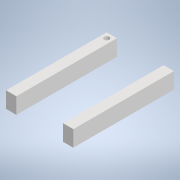
# Autodesk Inventor part: motor mount layer
Saved by Autodesk Inventor 2022 (Build 260153000, 153)
## iProperties
Created: 2021-11-30
Part Number: motor mount layer
Material: Generic
Document SubType Name: Modeling
Designer: a-dubs
Density: 1 g/cm^3
Appearance: Default
Author: a-dubs
Autodesk Inventor part; units mm, degrees
ref_plane "YZ Plane" through (0, 0, 0) normal (1, 0, 0) x (0, 1, 0)
ref_plane "XZ Plane" through (0, 0, 0) normal (0, 1, 0) x (-1, 0, 0)
ref_plane "XY Plane" through (0, 0, 0) normal (0, 0, 1) x (1, 0, 0)
sketch "Sketch1" plane through (0, 0, 0) normal (0, 1, 0) x (-1, 0, 0)
  line L0 (0, 0) -> (61, 0)
  circle A0 centre (0, 0) radius 33.6
  line L1 (61, 8.05) -> (61, 13.05)
  line L2 (72.05, 0) -> (77.05, 0)
  line L3 (61, 0) -> (61, 60)
  line L4 (0, 0) -> (-42.65, 0)
  line L5 (-42.65, 0) -> (-47.65, 0)
  line L6 (-47.65, 0) -> (-53.85, 0)
  line L7 (0, 0) -> (0, -33.6)
  line L8 (0, 0) -> (42.65, 0)
  line L9 (35.9999, 0) -> (29.9999, 0)
  line L10 (29.9999, 0) -> (29.9999, -31.3)
  line L11 (29.9999, -31.3) -> (29.9999, -37.5)
  line L12 (29.9999, -37.5) -> (78.3499, -37.5)
  line L13 (78.3499, 37.4) -> (29.9999, 37.4)
  line L14 (29.9999, 37.4) -> (29.9999, 0)
  line L15 (42.65, 31.2) -> (45.65, 31.2)
  line L16 (78.3499, 37.4) -> (82.5499, 37.4)
  line L17 (82.5499, 37.4) -> (82.5499, -37.5)
  line L18 (82.5499, -37.5) -> (78.3499, -37.5)
  line L19 (29.9999, 37.4) -> (36.3999, 37.4)
  line L20 (61, 0) -> (40, 0)
  line L21 (40, 0) -> (40, 37.4)
  line L22 (40, 0) -> (40, -37.5)
  line L23 (36.8, -37.4) -> (43.2, -37.4)
  line L24 (43.2, -37.4) -> (43.2, 37.4)
  line L25 (43.2, 37.4) -> (36.8, 37.4)
  line L26 (36.8, 37.4) -> (36.8, -37.4)
  line L27 (36.8, -37.4) -> (43.2, 37.4) construction
  line L28 (43.2, -37.4) -> (36.8, 37.4) construction
  line L29 (61, 0) -> (75.45, 0)
  line L30 (61, 0) -> (61, -18.5)
  line L31 (75.45, 18.5) -> (75.45, -18.5)
  line L32 (75.45, -18.5) -> (46.55, -18.5)
  line L33 (46.55, -18.5) -> (46.55, 18.5)
  line L34 (46.55, 18.5) -> (75.45, -18.5) construction
  line L35 (75.45, 18.5) -> (46.55, -18.5) construction
  line L36 (46.55, 18.5) -> (46.55, 37.4)
  line L37 (75.45, 18.5) -> (75.45, 37.4)
  line L38 (75.45, -18.5) -> (75.45, -37.5)
  line L39 (46.55, -18.5) -> (46.55, -37.5)
  line L40 (75.45, 18.5) -> (75.45, 28.1)
  circle A1 centre (75.45, 28.1) radius 1.6
  circle A2 centre (46.55, 28.1) radius 1.6
  line L41 (75.45, -18.5) -> (75.45, -28.1)
  circle A3 centre (75.45, -28.1) radius 1.6
  circle A4 centre (46.55, -28.1) radius 1.6
  line L42 (75.45, 28.1) -> (75.45, 31.3)
  line L43 (75.45, 31.3) -> (29.9999, 31.3)
  line L44 (75.45, -28.1) -> (75.45, -31.3)
  line L45 (75.45, -31.3) -> (29.9999, -31.3)
  line L46 (75.45, -28.1) -> (75.45, -24.9)
  line L47 (75.45, -24.9) -> (29.9999, -24.9)
  line L48 (46.55, 28.1) -> (40, 28.1)
  circle A5 centre (40, 28.1) radius 1.6
  line L49 (46.55, -28.1) -> (40, -28.1)
  circle A6 centre (40, -28.1) radius 1.6
  line L50 (75.45, 28.1) -> (75.45, 24.9)
  line L51 (75.45, 24.9) -> (29.9999, 24.9)
  line L52 (75.45, 31.3) -> (78.65, 31.3)
  line L53 (78.65, 31.3) -> (78.65, -31.3)
  line L54 (78.65, -31.3) -> (75.45, -31.3)
  line L55 (75.45, -31.3) -> (72.25, -31.3)
  line L56 (72.25, -31.3) -> (72.25, 31.3)
  line L57 (46.55, 28.1) -> (49.75, 28.1)
  line L58 (49.75, 31.3) -> (49.75, -37.5)
  circle A7 centre (75.45, -18.5) radius 1.6
  circle A8 centre (46.55, -18.5) radius 1.6
  line L59 (46.55, 18.5) -> (46.55, 21.7)
  line L60 (75.45, 18.5) -> (75.45, 13.7)
  line L61 (75.45, 13.7) -> (78.65, 13.7)
  line L62 (78.65, 13.7) -> (36.8, 13.7)
  line L63 (75.45, -18.5) -> (75.45, -21.7)
  line L64 (75.45, -21.7) -> (36.8, -21.7)
  line L65 (75.45, -21.7) -> (78.65, -21.7)
  line L66 (75.45, -18.5) -> (75.45, -13.7)
  line L67 (75.45, -13.7) -> (78.65, -13.7)
  line L68 (75.45, -13.7) -> (36.8, -13.7)
  line L69 (57.8, -13.7) -> (64.2, -13.7)
  line L70 (64.2, -13.7) -> (64.2, 13.7)
  line L71 (64.2, 13.7) -> (57.8, 13.7)
  line L72 (57.8, 13.7) -> (57.8, -13.7)
  line L73 (57.8, -13.7) -> (64.2, 13.7) construction
  line L74 (64.2, -13.7) -> (57.8, 13.7) construction
  line L75 (49.75, -3.2) -> (72.25, -3.2)
  line L76 (72.25, -3.2) -> (72.25, 3.2)
  line L77 (72.25, 3.2) -> (49.75, 3.2)
  line L78 (49.75, 3.2) -> (49.75, -3.2)
  line L79 (49.75, -3.2) -> (72.25, 3.2) construction
  line L80 (72.25, -3.2) -> (49.75, 3.2) construction
  line L81 (49.75, 3.2) -> (43.2, 3.2)
  line L82 (49.75, -3.2) -> (43.2, -3.2)
  line L83 (52.2, -8.45) -> (69.8, -8.45)
  line L84 (69.8, -8.45) -> (69.8, 8.45)
  line L85 (69.8, 8.45) -> (52.2, 8.45)
  line L86 (52.2, 8.45) -> (52.2, -8.45)
  line L87 (52.2, -8.45) -> (69.8, 8.45) construction
  line L88 (69.8, -8.45) -> (52.2, 8.45) construction
  line L89 (61, 0) -> (61, 22.2)
  line L90 (61, 22.2) -> (46.55, 22.2)
  line L91 (61, 22.2) -> (61, 17.4)
  line L92 (61, 17.4) -> (36.8, 17.4)
  line L93 (61, 22.2) -> (61, 25.4)
  line L94 (61, 25.4) -> (36.8, 25.4)
  line L95 (61, 25.4) -> (78.65, 25.4)
  line L96 (61, 17.4) -> (78.65, 17.4)
  line L97 (61, 22.2) -> (82.5499, 22.2)
  line L98 (46.55, 22.2) -> (36.8, 22.2)
  line L99 (61, 0) -> (61, -14.8)
  line L100 (61, -14.8) -> (61, -18)
  line L101 (61, -14.8) -> (61, -10)
  line L102 (61, -10) -> (36.8, -10)
  line L103 (61, -18) -> (36.8, -18)
  line L104 (61, -18) -> (82.5499, -18)
  line L105 (61, -10) -> (82.5499, -10)
  line L106 (64.2, 13.7) -> (64.2, 17.4)
  line L107 (57.8, 17.4) -> (57.8, 13.7)
  point P0 (36.8, 31.3)
  point P1 (36.8, -31.3)
  point P2 (43.2, -31.3)
  point P3 (43.2, 31.3)
  point P4 (43.2, -21.7)
  point P5 (72.25, -21.7)
  point P6 (43.2, 13.7)
  point P7 (72.25, 13.7)
  point P8 (72.25, -13.7)
  point P9 (43.2, -13.7)
  point P10 (57.8, -3.2)
  point P11 (64.2, -3.2)
  point P12 (64.2, 3.2)
  point P13 (57.8, 3.2)
  point P14 (57.8, 8.45)
  point P15 (64.2, 8.45)
  point P16 (52.2, -3.2)
  point P17 (52.2, 3.2)
  point P18 (61, 18.5)
  point P19 (72.25, 22.2)
  point P20 (46.55, 24.9)
  point P21 (43.2, 24.9)
  point P22 (43.2, 22.2)
  point P23 (72.25, -18)
  point P24 (72.25, -10)
  point P25 (64.2, -10)
  point P26 (64.2, -8.45)
  point P27 (57.8, -8.45)
  point P28 (57.8, -10)
  point P29 (43.2, -10)
  point P30 (43.2, -18)
  point P31 (72.25, 17.4)
  point P32 (72.25, 24.9)
  point P33 (43.2, 17.4)
  dimension "d1" = 67.2
  dimension "d0" = 61
  dimension "d7" = 5
  dimension "d8" = 5
  dimension "d11" = 60
  dimension "d13" = 42.65
  dimension "d14" = 5
  dimension "d15" = 6.2
  dimension "d26" = 6
  dimension "d27" = 6.2
  dimension "d42" = 3
  dimension "d46" = 4.2
  dimension "d53" = 6.4
  dimension "d54" = 21
  dimension "d55" = 6.4
  dimension "d56" = 14.45
  dimension "d57" = 18.5
  dimension "d58" = 9.6
  dimension "d60" = 3.2
  dimension "d61" = 3.2
  dimension "d62" = 3.2
  dimension "d63" = 3.2
  dimension "d64" = 3.2
  dimension "d66" = 3.2
  dimension "d67" = 3.2
  dimension "d68" = 3.2
  dimension "d69" = 3.2
  dimension "d70" = 3.2
  dimension "d71" = 3.2
  dimension "d74" = 3.2
  dimension "d75" = 3.2
  dimension "d78" = 3.2
  dimension "d79" = 4.8
  dimension "d80" = 3.2
  dimension "d81" = 4.8
  dimension "d85" = 6.4
  dimension "d86" = 6.4
  dimension "d87" = 17.6
  dimension "d88" = 16.9
  dimension "d89" = 22.2
  dimension "d90" = 4.8
  dimension "d91" = 3.2
  dimension "d92" = 14.8
  dimension "d93" = 3.2
  dimension "d94" = 4.8
  constraints: 214 end point, 65 point on line, 29 perpendicular, 18 horizontal, 11 coincident, 10 midpoint, 10 parallel, 8 centre point, 6 vertical, 4 symmetric about line, 1 vertical alignment, 15 other
  measures "d0" distance of L0.start L0.end
  measures "d7" distance of L1.start L1.end
  measures "d8" distance of L2.start L2.end
  measures "d11" distance of L3.start L3.end
  measures "d13" distance of L4.start L4.end
  measures "d14" distance of L4.end L5.end
  measures "d15" distance of L5.end L6.end
  measures "d26" distance of L9.start L9.end
  measures "d27" distance of L10.end L11.end
  measures "d42" distance of L15.start L15.end
  measures "d46" distance of L13.start L16.end
  measures "d53" distance of L13.end L19.end
  measures "d54" distance of L20.start L20.end
  measures "d55" distance of L25.end L24.end
  measures "d56" distance of L20.start L29.end
  measures "d57" distance of L20.start L30.end
  measures "d58" distance of L31.start L40.end
  measures "d60" diameter of A1
  measures "d61" diameter of A2
  measures "d62" distance of L42.start L42.end
  measures "d63" distance of L44.start L44.end
  measures "d64" distance of L44.start L46.end
  measures "d66" diameter of A5
  measures "d67" diameter of A6
  measures "d68" distance of L42.start L50.end
  measures "d69" distance of L42.end L52.end
  measures "d70" distance of L44.end L55.end
  measures "d71" distance of L48.start L57.end
  measures "d74" diameter of A7
  measures "d75" diameter of A8
  measures "d78" distance of L59.start L59.end
  measures "d79" distance of L60.start L60.end
  measures "d80" distance of L63.start L63.end
  measures "d81" distance of L63.start L66.end
  measures "d85" distance of L71.end L70.end
  measures "d86" distance of L76.end L75.end
  measures "d87" distance of L85.end L84.end
  measures "d88" distance of L84.end L83.end
  measures "d89" distance of L20.start L89.end
  measures "d90" distance of L89.end L91.end
  measures "d91" distance of L89.end L93.end
  measures "d92" distance of L20.start L99.end
  measures "d93" distance of L99.end L100.end
  measures "d94" distance of L99.end L101.end
extrude "Extrusion2" add sketch "Sketch1" along normal blind 6.4 contours L26 L62 L21 L0 | L0 L22 L102 L26 | L47 L22 A6 L45 L26 | L26 L64 L22 L47 | L51 L21 L98 L26 | L26 L94 L21 L51 | L21 L62 L24 L0 | L0 L24 L102 L22 | L26 L92 L21 L62 | L102 L22 L68 L26 | L26 L103 L22 L64 | L47 L24 L49 A6 L22 | L22 L64 L24 L47 | L43 L21 A5 L94 L26 | L98 L21 L92 L26 | L51 L24 L98 L21 | L21 L94 L24 L51 | L21 L92 L24 L62 | L102 L24 L68 L22 | L68 L22 L103 L26 | L22 A6 L49 L24 L45 | L22 L103 L24 L64 | L43 L24 L48 A5 L21 | L21 A5 L48 L24 L94 | L98 L24 L92 L21 | L51 L36 L98 L24 | L24 L81 L33 L0 | L0 L33 L82 L24 | L68 L24 L103 L22 | L102 L33 L68 L24 | L98 L36 L33 L92 L24 | L51 L58 L90 L36 | L33 L81 L58 L0 | L0 L58 L82 L33 | L68 L33 A8 L103 L24 | L102 L58 L68 L33 | L90 L58 L92 L33 L36 | L51 L3 L90 L58 | L58 L77 L86 L0 | L0 L86 L75 L58 | L68 L58 L103 A8 L33 | L102 L72 L68 L58 | A8 L33 L103 | L56 L64 L38 L47 | L47 L38 A3 L45 L56 | L90 L3 L92 L58 | L51 L56 L97 L3 | L107 L92 L3 L62 | L62 L3 L1 L85 L72 | A8 L103 L33 | L68 L30 L103 L58 | L102 L30 L68 L72 | L72 L83 L30 L102 | L38 A3 L65 L53 L54 | L56 L32 A7 L38 L64 | L97 L56 L96 L3 | L56 L95 L37 L51 | L51 L37 L97 L56 | L62 L70 L85 L1 L3 | L3 L96 L106 L62 | L105 L70 L68 L30 | L30 L83 L70 L105 | L56 L104 A7 L32 | L38 A7 L104 L53 L65 | L43 L37 A1 L95 L56 | L97 L37 L31 L96 L56 | L37 L95 L53 L97 | L30 L68 L56 L104 | L105 L56 L68 L70 | A7 L104 L31 L32 | L32 L38 A7 | L56 L68 L31 A7 L104 | L38 L31 L104 A7 | L52 L53 L95 L37 A1 | L96 L31 L62 L56 | L97 L53 L96 L31 L37 | L62 L31 L2 L56 | L105 L31 L68 L56 | L56 L2 L31 L105 | L104 A7 L31 L67 L53 | A7 L31 L104 | L96 L53 L61 L31 | L61 L53 L105 L31 | L105 L53 L67 L31 | L104 L31 A7
chamfer "Chamfer3" distance 1.6 angle 45 32 edges at (-40, 6.4, 31.3) (-36.8, 6.4, 0) (-43.2, 6.4, -6.6) (-43.2, 6.4, -24.65) (-43.2, 6.4, 10.3) (-43.2, 6.4, 28.1) (-40, 6.4, -31.3) (-72.25, 6.4, 3.7) (-72.25, 6.4, -24.65) (-72.25, 6.4, 28.1) (-78.65, 6.4, 0) (-75.45, 6.4, 31.3) (-47.7, 6.4, 3.2) (-57.8, 6.4, -9.225) (-64.2, 6.4, -9.225) (-47.7, 6.4, -3.2) (-50.5, 6.4, -10) (-57.725, 6.4, -18) (-68.225, 6.4, -10) (-78.65, 3.2, -31.3) (-72.25, 3.2, -31.3) (-43.2, 3.2, -31.3) (-36.8, 3.2, -31.3) (-78.65, 3.2, 31.3) (-72.25, 3.2, 31.3) (-43.2, 3.2, 31.3) (-36.8, 3.2, 31.3) (-68.225, 6.4, 17.4) (-50.5, 6.4, 17.4) (-57.725, 6.4, 24.9) (-57.8, 6.4, 12.925) (-64.2, 6.4, 12.925)
body "Solid2"
